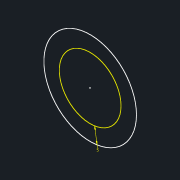
# Autodesk Inventor part: spline Hub
Saved by Autodesk Inventor 2021 (Build 250183000, 183)
## iProperties
Created: 2020-10-16
Part Number: spline Hub
Material: Generic
Document SubType Name: Modeling
Designer: Eugene Tang
Mass: 19.635 g
Surface Area: 86.3938 cm^2
Volume: 19.635 cm^3
Density: 1 g/cm^3
Appearance: Default
Author: Eugene Tang
Autodesk Inventor part; units mm, degrees
ref_plane "YZ Plane" through (0, 0, 0) normal (1, 0, 0) x (0, 1, 0)
ref_plane "XZ Plane" through (0, 0, 0) normal (0, 1, 0) x (-1, 0, 0)
sketch "Sketch1" plane through (0, 0, 0) normal (0, 0, 1) x (1, 0, 0)
  circle A0 centre (0, 0) radius 10 projected
  circle A1 centre (0, 0) radius 15
  dimension "d0" = 5
  constraints: 1 centre point, 1 coincident
  measures "d0" radial gap between concentric circles of A1 A0
ref_plane "Work Plane1" through (-11.1146, -11.1146, 50) normal (0, 0, 1) x (1, 0, 0)
extrude "Extrusion1" add sketch "Sketch1" along normal up to surface (50 mm away)
body "Solid1"
